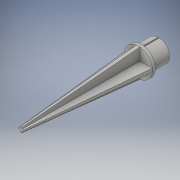
# Autodesk Inventor part: GroundSupport
Saved by Autodesk Inventor 2016 SP1 (Build 200210100, 210)
## iProperties
Created: 2015-11-21
Part Number: GroundSupport
Material: Generic
Document SubType Name: Modeling
Designer: steele
Density: 1 g/cm^3
Appearance: Default
Author: steele
Autodesk Inventor part; units mm, degrees
ref_plane "YZ Plane" through (0, 0, 0) normal (1, 0, 0) x (0, 1, 0)
ref_plane "XZ Plane" through (0, 0, 0) normal (0, 1, 0) x (-1, 0, 0)
ref_plane "XY Plane" through (0, 0, 0) normal (0, 0, 1) x (1, 0, 0)
sketch "Sketch1" plane through (0, 0, 0) normal (0, 0, 1) x (1, 0, 0)
  circle A0 centre (0, 0) radius 15.24
  dimension "d0" = 30.48
  constraints: 1 centre point, 1 coincident
  measures "d0" diameter of A0
extrude "Extrusion1" add sketch "Sketch1" along normal mid plane 3.175
sketch "Sketch2" plane through (0, 0, -1.5875) normal (0, 0, -1) x (-1, 0, 0)
  circle A0 centre (0, 0) radius 11.938
  dimension "d3" = 23.876
  constraints: 1 centre point, 1 coincident
  measures "d3" diameter of A0
extrude "Extrusion2" add sketch "Sketch2" along normal blind 19.05
sketch "Sketch4" plane through (0, 0, 1.5875) normal (0, 0, 1) x (1, 0, 0)
  line L0 (-15.24, 1.905) -> (-15.24, -1.905)
  line L1 (-15.24, -1.905) -> (-1.905, -1.905)
  line L2 (-1.905, -1.905) -> (-1.905, -15.24)
  line L3 (-1.905, -15.24) -> (1.905, -15.24)
  line L4 (1.905, -15.24) -> (1.905, -1.905)
  line L5 (1.905, -1.905) -> (15.24, -1.905)
  line L6 (15.24, -1.905) -> (15.24, 1.905)
  line L7 (15.24, 1.905) -> (1.905, 1.905)
  line L8 (1.905, 1.905) -> (1.905, 15.24)
  line L9 (1.905, 15.24) -> (-1.905, 15.24)
  line L10 (-1.905, 15.24) -> (-1.905, 1.905)
  line L11 (-1.905, 1.905) -> (-15.24, 1.905)
  line L12 (-15.2163, 0) -> (15.24, 0) construction
  circle A0 centre (0, 0) radius 15.24 construction
  line L13 (0.0118, 15.24) -> (0, -15.24) construction
  dimension "d7" = 15.24
  dimension "d8" = 15.24
  dimension "d31" = 3.81
  dimension "d10" = 1.905
  dimension "d11" = 3.81
  constraints: 28 end point, 11 perpendicular, 4 point on line, 3 point on circle, 2 parallel, 1 collinear, 1 horizontal, 1 vertical
  measures "d7" distance from line of L0 point (0, 0)
  measures "d8" distance from line of point (0, 0) L9
  measures "d31" distance of L8.end L9.end
  measures "d10" distance from line of point (0, 0) L8
  measures "d11" distance of L0.start L0.end
ref_plane "Work Plane1" through (0, 0, 128.5875) normal (0, 0, 1) x (1, 0, 0)
sketch "Sketch5" plane through (0, 0, 128.5875) normal (0, 0, 1) x (1, 0, 0)
  line L0 (-0.8467, 2.54) -> (-0.8467, 0.8467)
  line L1 (-0.8467, 0.8467) -> (-2.54, 0.8467)
  line L2 (-2.54, 0.8467) -> (-2.54, -0.8467)
  line L3 (-2.54, -0.8467) -> (-0.8467, -0.8467)
  line L4 (-0.8467, -0.8467) -> (-0.8467, -2.54)
  line L5 (-0.8467, -2.54) -> (0.8467, -2.54)
  line L6 (0.8467, -2.54) -> (0.8467, -0.8467)
  line L7 (0.8467, -0.8467) -> (2.54, -0.8467)
  line L8 (2.54, -0.8467) -> (2.54, 0.8467)
  line L9 (2.54, 0.8467) -> (0.8467, 0.8467)
  line L10 (0.8467, 2.54) -> (-0.8467, 2.54)
  line L11 (0.8467, 2.54) -> (0.8467, 0.8467)
  point P0 (0, 0)
  dimension "d23" = 1.6933
  dimension "d24" = 0.8467
  dimension "d25" = 0.8467
  dimension "d26" = 5.08
  dimension "d27" = 2.54
  dimension "d28" = 2.54
  dimension "d29" = 5.08
  dimension "d30" = 1.6933
  constraints: 24 end point, 8 point on line, 7 perpendicular, 1 parallel, 1 vertical
  measures "d23" distance between parallel lines of L6 L4
  measures "d24" distance from line of L6 point (0, 0)
  measures "d25" distance from line of L7 point (0, 0)
  measures "d26" distance between parallel lines of L10 L5
  measures "d27" distance from line of L10 point (0, 0)
  measures "d28" distance from line of L8 point (0, 0)
  measures "d29" distance between parallel lines of L2 L8
  measures "d30" distance of L1.end L2.end
loft "Loft1" add profiles "Sketch5", "Sketch4"
sketch "Sketch6" plane through (0, 0, -20.6375) normal (0, 0, -1) x (-1, 0, 0)
  line L0 (-13.208, -0.635) -> (13.208, -0.635)
  line L1 (13.208, -0.635) -> (13.208, 0.635)
  line L2 (13.208, 0.635) -> (-13.208, 0.635)
  line L3 (-13.208, 0.635) -> (-13.208, -0.635)
  line L4 (-13.208, -0.635) -> (13.208, 0.635) construction
  line L5 (13.208, -0.635) -> (-13.208, 0.635) construction
  line L6 (-0.635, 13.208) -> (-0.635, -13.208)
  line L7 (-0.635, -13.208) -> (0.635, -13.208)
  line L8 (0.635, -13.208) -> (0.635, 13.208)
  line L9 (0.635, 13.208) -> (-0.635, 13.208)
  line L10 (-0.635, 13.208) -> (0.635, -13.208) construction
  line L11 (-0.635, -13.208) -> (0.635, 13.208) construction
  point P0 (0, 0)
  dimension "d18" = 1.27
  dimension "d19" = 26.416
  constraints: 24 end point, 4 midpoint, 4 parallel, 4 perpendicular, 1 horizontal, 1 vertical
  measures "d18" distance of L0.end L1.end
  measures "d19" distance of L0.start L0.end
extrude "Extrusion3" cut sketch "Sketch6" against normal blind 16.51
equation "\"d0\" = outerDiam"
equation "\"d1\" = supportThickness"
equation "\"d3\" = lightSupportDiam"
equation "\"d4\" = lightSupportLength"
equation "\"d7\" = 0.5 * outerDiam"
equation "\"d8\" = 0.5 * outerDiam"
equation "\"d31\" = vaneThickness"
equation "\"d10\" = 0.5 * vaneThickness"
equation "\"d11\" = vaneThickness"
equation "\"d23\" = 0.333333 * vaneEndDiam"
equation "\"d24\" = 0.166667 * vaneEndDiam"
equation "\"d25\" = 0.166667 * vaneEndDiam"
equation "\"d26\" = vaneEndDiam"
equation "\"d27\" = 0.5 * vaneEndDiam"
equation "\"d28\" = 0.5 * vaneEndDiam"
equation "\"d29\" = vaneEndDiam"
equation "\"d30\" = 0.333333 * vaneEndDiam"
equation "\"d18\" = lightSlotWidth"
equation "\"d19\" = lightSlotLength"
equation "\"d20\" = lightSlotDepth"
equation "\"outerDiam\" = 30.48"
equation "\"supportThickness\" = 3.175"
equation "\"lightSupportDiam\" = 23.876"
equation "\"lightSupportLength\" = 19.05"
equation "\"groundLength\" = 127"
equation "\"d12\" = groundLength"
equation "\"lightSlotWidth\" = 1.27"
equation "\"vaneEndDiam\" = 5.08"
equation "\"vaneThickness\" = 3.81"
equation "\"lightSlotLength\" = 26.416"
equation "\"lightSlotDepth\" = 16.51"
body "Solid1"
